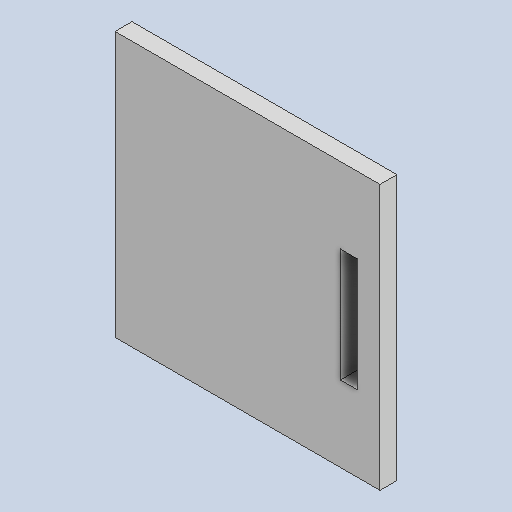
# Autodesk Inventor part: pcb
Saved by Autodesk Inventor 2022 (Build 260153000, 153)
## iProperties
Created: 2023-01-18
Part Number: pcb
Material: Generic
Document SubType Name: Modeling
Designer: komputer
Density: 1 g/cm^3
Appearance: Default
Author: komputer
Autodesk Inventor part; units mm, degrees
ref_plane "YZ Plane" through (0, 0, 0) normal (1, 0, 0) x (0, 1, 0)
ref_plane "XZ Plane" through (0, 0, 0) normal (0, 1, 0) x (-1, 0, 0)
ref_plane "XY Plane" through (0, 0, 0) normal (0, 0, 1) x (1, 0, 0)
sketch "Sketch1" plane through (0, 0, 0) normal (0, 0, 1) x (1, 0, 0)
  line L0 (-11.2628, -8.9945) -> (-11.2628, -13.0945)
  line L1 (-11.2628, 11.9772) -> (-11.2628, 7.8772)
  line L2 (12.7, 5.5055) -> (12.7, -0.323) projected
  line L3 (12.7, -6.6945) -> (-7.3, -6.6945)
  line L4 (12.7, 5.5055) -> (-7.3, 5.5055)
  line L5 (-10.4, -1.4801) -> (-10.4, -2.591) projected
  line L6 (-10.4, 0.291) -> (-10.4, 1.4019) projected
  line L7 (12.7, -6.6945) -> (-10.4, -6.6945)
  line L8 (-10.4, -6.6945) -> (-10.4, 5.5055)
  line L9 (-10.4, 5.5055) -> (12.7, 5.5055)
  line L10 (12.7, 5.5055) -> (12.7, -6.6945)
  line L11 (12.7, 5.5055) -> (-11.2628, 5.5055)
  line L12 (-11.2628, 5.5055) -> (-11.2628, -6.6945)
  line L13 (-11.2628, -6.6945) -> (12.7, -6.6945)
  line L14 (12.7, -6.6945) -> (12.7, 5.5055)
  line L15 (-11.2628, -0.5945) -> (-12.5719, -0.5945)
  line L16 (-11.2628, -0.5945) -> (13.7372, -0.5945)
  line L17 (13.7372, -0.5945) -> (13.7372, -13.0945)
  line L18 (13.7372, -13.0945) -> (-11.2628, -13.0945)
  line L19 (-11.2628, -13.0945) -> (-11.2628, -0.5945)
  line L20 (13.7372, -0.5945) -> (13.7372, 11.9055)
  line L21 (13.7372, 11.9055) -> (-11.2628, 11.9055)
  line L22 (-11.2628, 11.9055) -> (-11.2628, -0.5945)
  line L23 (11.6, -5.6608) -> (10, -5.6608) projected
  line L24 (11.6, 5.0392) -> (10, 5.0392) projected
  line L25 (11.6, 5.0392) -> (11.6, -5.6608) projected
  line L26 (11.6, 5.0392) -> (10, 5.0392) projected
  line L27 (10, -5.6608) -> (10, 5.0392) projected
  line L28 (11.6, -5.6608) -> (10, -5.6608) projected
  line L29 (11.6, -0.5945) -> (11.6, -5.9445)
  line L30 (11.6, -5.9445) -> (10, -5.9445)
  line L31 (10, -5.9445) -> (10, -0.5945)
  line L32 (11.6, -0.5945) -> (11.6, 4.7555)
  line L33 (11.6, 4.7555) -> (10, 4.7555)
  line L34 (10, 4.7555) -> (10, -0.5945)
  point P0 (0, 0)
  point P1 (-11.2628, -6.6945)
  dimension "d2" = 23.9628
  dimension "d3" = 25
  dimension "d4" = 12.5
  dimension "d5" = 5.35
  constraints: 52 end point, 6 horizontal, 6 parallel, 5 point on line, 4 perpendicular, 4 symmetric about line, 2 vertical, 1 midpoint, 7 other
  measures "d2" distance of L9.end L11.end
  measures "d3" distance of L17.end L18.end
  measures "d4" distance of L16.end L17.end
  measures "d5" distance of L29.start L29.end
extrude "Extrusion1" add sketch "Sketch1" along normal blind 1.6 contours L19 L13 L7 L3 L10 L16 L17 L18 L0 | L12 L16 L8 L5 L13 | L12 L11 L8 L6 L16 | L8 L5 L16 L27 L31 L30 L29 L25 L10 L3 L7 | L16 L10 L2 L4 L9 L11 L22 L1 L21 L20 | L8 L6 L9 L4 L2 L10 L16 L25 L24 L27 | L27 L24 L25 L33
body "Solid1"
